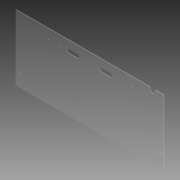
# Autodesk Inventor part: FE-120-009 Door Panel
Saved by Autodesk Inventor 2021 (Build 250183000, 183)
## iProperties
Created: 2021-01-12
Part Number: FE-120-009 Door Panel
Material: Polycarbonate, Clear
Document SubType Name: Modeling
Density: 1.2 g/cm^3
Appearance: Polycarbonate - Clear
Autodesk Inventor part; units mm, degrees
ref_plane "YZ Plane" through (0, 0, 0) normal (1, 0, 0) x (0, 1, 0)
ref_plane "XZ Plane" through (0, 0, 0) normal (0, 1, 0) x (-1, 0, 0)
ref_plane "XY Plane" through (0, 0, 0) normal (0, 0, 1) x (1, 0, 0)
sketch "Sketch1" plane through (0, 0, 0) normal (0, 0, 1) x (1, 0, 0)
  line L0 (-571.5, -254) -> (571.5, -254)
  line L1 (571.5, -254) -> (571.5, 254)
  line L2 (571.5, 254) -> (-571.5, 254)
  line L3 (-571.5, 254) -> (-571.5, -254)
  line L4 (-571.5, -254) -> (571.5, 254) construction
  line L5 (571.5, -254) -> (-571.5, 254) construction
  line L6 (-158.75, 180.975) -> (-95.25, 180.975) construction
  line L7 (-158.75, 165.1) -> (-95.25, 165.1)
  line L8 (-95.25, 196.85) -> (-158.75, 196.85)
  arc A0 (-158.75, 196.85) -> (-158.75, 165.1) centre (-158.75, 180.975) ccw
  arc A1 (-95.25, 165.1) -> (-95.25, 196.85) centre (-95.25, 180.975) ccw
  line L9 (95.25, 180.975) -> (158.75, 180.975) construction
  line L10 (95.25, 165.1) -> (158.75, 165.1)
  line L11 (158.75, 196.85) -> (95.25, 196.85)
  arc A2 (95.25, 196.85) -> (95.25, 165.1) centre (95.25, 180.975) ccw
  arc A3 (158.75, 165.1) -> (158.75, 196.85) centre (158.75, 180.975) ccw
  line L12 (485.775, 266.7) -> (485.775, 241.3) construction
  line L13 (466.725, 266.7) -> (466.725, 241.3)
  line L14 (504.825, 241.3) -> (504.825, 266.7)
  arc A4 (504.825, 266.7) -> (466.725, 266.7) centre (485.775, 266.7) ccw construction
  arc A5 (466.725, 241.3) -> (504.825, 241.3) centre (485.775, 241.3) ccw
  point P0 (0, 0)
  point P1 (-127, 180.975)
  point P2 (127, 180.975)
  point P3 (485.775, 254)
  point P4 (504.825, 254)
  point P5 (466.725, 254)
  dimension "d0" = 1143
  dimension "d1" = 508
  dimension "d2" = 15.875
  dimension "d3" = 63.5
  dimension "d4" = 190.5
  dimension "d5" = 95.25
  dimension "d6" = 57.15
  dimension "d7" = 38.1
  dimension "d8" = 12.7
  dimension "d9" = 66.675
  constraints: 36 end point, 12 point on circle, 12 tangent, 7 parallel, 6 centre point, 5 midpoint, 2 collinear, 2 perpendicular, 1 equal radius, 1 horizontal, 1 point on line
  measures "d0" distance of L2.end L1.end
  measures "d1" distance of L1.end L0.end
  measures "d2" radius of A2
  measures "d3" distance of L9.start L9.end
  measures "d4" distance of L6.end L9.start
  measures "d5" horizontal distance of point (0, 0) L6.end
  measures "d6" distance between parallel lines of L2 L8
  measures "d7" diameter of A5
  measures "d8" distance from line of L12.end L2
  measures "d9" distance between parallel lines of L1 L14
extrude "Extrusion1" add sketch "Sketch1" along normal blind 6.35 contours L3 L2 L13 A5 L14 L1 L0
sketch "Sketch2" plane through (0, 0, 6.35) normal (0, 0, 1) x (1, 0, 0)
  arc A0 (-158.75, 196.85) -> (-158.75, 165.1) centre (-158.75, 180.975) ccw construction
  arc A1 (158.75, 165.1) -> (158.75, 196.85) centre (158.75, 180.975) ccw construction
  line L0 (-571.5, 254) -> (-571.5, -254) construction
  line L1 (-571.5, -254) -> (571.5, -254) construction
  line L2 (571.5, -254) -> (571.5, 254) construction
  point P0 (0, 0)
  point P1 (-323.85, 180.975)
  point P2 (-222.25, 180.975)
  point P3 (222.25, 180.975)
  point P4 (323.85, 180.975)
  point P5 (-549.275, -165.1)
  point P6 (-530.225, -146.05)
  point P7 (530.225, -165.1)
  point P8 (549.275, -146.05)
  dimension "d12" = 101.6
  dimension "d13" = 63.5
  dimension "d14" = 101.6
  dimension "d15" = 63.5
  dimension "d17" = 19.05
  dimension "d18" = 19.05
  dimension "d20" = 88.9
  dimension "d22" = 22.225
  dimension "d30" = 19.05
  dimension "d31" = 22.225
  constraints: 6 horizontal alignment
  measures "d12" distance of point (-222.25, 180.975) point (-323.85, 180.975)
  measures "d13" distance of A0.centre point (-222.25, 180.975)
  measures "d14" distance of point (323.85, 180.975) point (222.25, 180.975)
  measures "d15" distance of point (222.25, 180.975) A1.centre
  measures "d17" horizontal distance of point (-549.275, -165.1) point (-530.225, -146.05)
  measures "d18" horizontal distance of point (549.275, -146.05) point (530.225, -165.1)
  measures "d20" distance from line of L1 point (-549.275, -165.1)
  measures "d22" distance from line of point (549.275, -146.05) L2
  measures "d30" horizontal distance of point (-530.225, -146.05) point (-549.275, -165.1)
  measures "d31" distance from line of L0 point (-549.275, -165.1)
hole "Hole1" at (-323.85, 180.975, 6.35) at (-222.25, 180.975, 6.35) at (222.25, 180.975, 6.35) at (323.85, 180.975, 6.35) at (-549.275, -165.1, 6.35) at (-530.225, -146.05, 6.35) at (530.225, -165.1, 6.35) at (549.275, -146.05, 6.35) direction (0, 0, -1) diameter 6.35 end through all countersink diameter 13.1064 countersink angle 82
equation "\"d5\" = 0.5 * d4"
equation "\"d14\" = d12"
equation "\"d15\" = d13"
equation "\"d18\" = d16"
equation "\"d16\" = 19.05"
body "Solid1"
